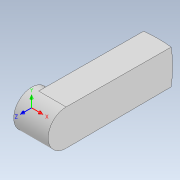
# Autodesk Inventor part: shank_inventor
Saved by Autodesk Inventor 2020 (Build 240168000, 168)
## iProperties
Created: 2021-01-07
Part Number: shank_inventor
Material: Generic
Document SubType Name: Modeling
Designer: DELL
Density: 1 g/cm^3
Appearance: Default
Author: DELL
Autodesk Inventor part; units mm, degrees
ref_plane "YZ Plane" through (0, 0, 0) normal (1, 0, 0) x (0, 1, 0)
ref_plane "XY Plane" through (0, 0, 0) normal (0, 0, 1) x (1, 0, 0)
ref_plane "UCS1: YZ Plane" through (0, 0, 0) normal (1, 0, 0) x (0, 1, 0)
sketch "Sketch2" plane through (0, 0, 0) normal (1, 0, 0) x (0, 1, 0)
  circle A0 centre (0, 0) radius 26
  line L0 (25, -156) -> (-25, -156)
  line L1 (0, 0) -> (0, -156) construction
  line L2 (-25.9995, -0.1668) -> (-25, -156)
  line L3 (25.9995, -0.1668) -> (25, -156)
  dimension "d1" = 52
  dimension "d3" = 50
  dimension "d20" = 156
  constraints: 8 end point, 2 point on circle, 1 centre point, 1 coincident, 1 horizontal, 1 midpoint, 1 perpendicular, 1 tangent, 1 other
  measures "d1" diameter of A0
  measures "d3" distance of L0.start L0.end
  measures "d20" distance from line of point (0, 0) L0
extrude "Extrusion1" add sketch "Sketch2" along normal blind 50 contours A0
extrude "Extrusion2" add sketch "Sketch2" against normal blind 40 from surface at 50 contours A0 L3 L0 L2
sketch "Sketch5" plane through (50, -25, -156) normal (0, 0, -1) x (-1, 0, 0)
  circle A0 centre (20, 25) radius 10
  line L0 (40, 50) -> (0, 50) projected
  line L1 (40, 50) -> (40, 0) projected
  point P0 (50, 25)
  point P1 (20, 50)
  point P2 (40, 25)
  dimension "d22" = 20
  constraints: 2 midpoint, 1 centre point, 1 horizontal alignment, 1 vertical alignment
  measures "d22" diameter of A0
extrude "Extrusion4" cut sketch "Sketch5" against normal blind 60
ref_plane "Work Plane1" through (30, 0, 0) normal (-1, 0, 0) x (0, 0, -1)
sketch "Sketch4" plane through (30, 0, 0) normal (-1, 0, 0) x (0, 0, -1)
  line L0 (156, -25) -> (156, 25) projected
  arc A0 (150.7846, -40) -> (156, 0) centre (0, 0) ccw
  line L1 (150.7846, -40) -> (156, -40)
  line L2 (156, -40) -> (156, 0)
  line L3 (-62.6597, 0) -> (193.958, 0) projected
  line L4 (0, 0) -> (156, 0)
  dimension "d18" = 40
  constraints: 6 end point, 2 horizontal, 2 point on circle, 1 centre point, 1 coincident, 1 midpoint, 1 perpendicular
  measures "d18" distance between parallel lines of L3 L1
revolve "Revolution1" cut sketch "Sketch4" angle 360 about axis through (30, 0, 0) along (0, 0, -1)
body "Solid1"
